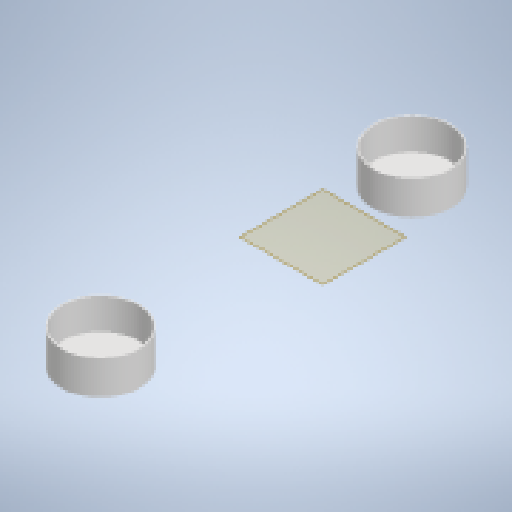
# Autodesk Inventor part: Base
Saved by Autodesk Inventor 2023.1 (Build 271208000, 208)
## iProperties
Created: 2023-07-08
Part Number: Base
Material: Generic
Document SubType Name: Modeling
Designer: Robot
Density: 1 g/cm^3
Appearance: Default
Author: Robot
Autodesk Inventor part; units mm, degrees
ref_plane "YZ Plane" through (0, 0, 0) normal (1, 0, 0) x (0, 1, 0)
ref_plane "XZ Plane" through (0, 0, 0) normal (0, 1, 0) x (-1, 0, 0)
ref_plane "XY Plane" through (0, 0, 0) normal (0, 0, 1) x (1, 0, 0)
ref_plane "Work Plane1" through (-8.7385, 18226.0351, -280.5199) normal (0, 1, 0) x (-0.9985279, 0, -0.0542412)
sketch "Sketch1" plane through (-8.7385, 18226.0351, -280.5199) normal (0, 1, 0) x (-0.9985279, 0, -0.0542412)
  circle A0 centre (-0.1598, -60.199) radius 25.4
  circle A1 centre (-0.1598, 150.601) radius 25.4
  circle A2 centre (-0.1598, 150.601) radius 26.4
  circle A3 centre (-0.1598, -60.199) radius 26.4
  line L0 (-17.3085, -5.3414) -> (16.6915, -5.3414)
  line L1 (16.6915, -5.3414) -> (16.6915, 52.8634)
  line L2 (16.6915, 52.8634) -> (-17.3085, 52.8634)
  line L3 (-17.3085, 52.8634) -> (-17.3085, -5.3414)
  line L4 (-17.3085, 52.8634) -> (-17.3085, 130.529)
  line L5 (-17.3085, -5.3414) -> (-17.3085, -40.1271)
  line L6 (16.6915, -5.3414) -> (16.6915, -39.8768)
  line L7 (16.6915, 52.8634) -> (16.6915, 130.2787)
  line L8 (31.4252, -66.238) -> (7.3835, -90.2796)
  line L9 (7.3835, -90.2796) -> (61.8308, -144.7269)
  line L10 (61.8308, -144.7269) -> (85.8724, -120.6852)
  line L11 (85.8724, -120.6852) -> (31.4252, -66.238)
  line L12 (30.0109, -67.6522) -> (84.4582, -122.0994)
  line L13 (8.7977, -88.8654) -> (63.245, -143.3126)
  line L14 (-6.1639, -91.881) -> (-30.2055, -67.8394)
  line L15 (-30.2055, -67.8394) -> (-84.6528, -122.2866)
  line L16 (-84.6528, -122.2866) -> (-60.6111, -146.3283)
  line L17 (-60.6111, -146.3283) -> (-6.1639, -91.881)
  line L18 (-7.5781, -90.4668) -> (-62.0253, -144.914)
  line L19 (-28.7913, -69.2536) -> (-83.2386, -123.7008)
  line L20 (84.9349, 211.9974) -> (60.8933, 236.039)
  line L21 (60.8933, 236.039) -> (6.446, 181.5918)
  line L22 (6.446, 181.5918) -> (30.4877, 157.5502)
  line L23 (30.4877, 157.5502) -> (84.9349, 211.9974)
  line L24 (83.5207, 213.4116) -> (29.0735, 158.9644)
  line L25 (62.3075, 234.6248) -> (7.8603, 180.1776)
  line L26 (-32.1213, 155.9317) -> (-8.0796, 179.9733)
  line L27 (-86.5685, 210.3789) -> (-32.1213, 155.9317)
  line L28 (-85.1543, 211.7931) -> (-30.707, 157.3459)
  line L29 (-62.5268, 234.4205) -> (-86.5685, 210.3789)
  line L30 (-63.9411, 233.0063) -> (-9.4938, 178.5591)
  line L31 (-8.0796, 179.9733) -> (-62.5268, 234.4205)
  line L32 (-7.5781, -90.4668) -> (-3.4984, -86.3871)
  line L33 (-6.1639, -91.881) -> (-0.8723, -86.5894)
  line L34 (-30.2055, -67.8394) -> (-26.295, -63.9289)
  line L35 (-28.7913, -69.2536) -> (-25.8437, -66.306)
  line L36 (31.4252, -66.238) -> (26.2268, -61.0397)
  line L37 (30.0109, -67.6522) -> (26.0131, -63.6544)
  line L38 (8.7977, -88.8654) -> (5.8404, -85.9081)
  line L39 (7.3835, -90.2796) -> (3.1788, -86.3871)
  line L40 (29.0735, 158.9644) -> (25.7539, 155.6448)
  line L41 (30.4877, 157.5502) -> (26.1142, 153.1768)
  line L42 (7.8603, 180.1776) -> (4.3036, 176.6209)
  line L43 (6.446, 181.5918) -> (1.7836, 176.9293)
  line L44 (-8.0796, 179.9733) -> (-4.7119, 176.6056)
  line L45 (-9.4938, 178.5591) -> (-7.0269, 176.0922)
  line L46 (-30.707, 157.3459) -> (-26.443, 153.0818)
  line L47 (-32.1213, 155.9317) -> (-26.5588, 150.3692)
  point P0 (-23.9414, 279.6329)
  point P1 (-30.2055, -67.8394)
  dimension "d3" = 52.8
  dimension "d4" = 52.8
  dimension "d0" = 50.8
  dimension "d1" = 50.8
  dimension "d2" = 210.8
  dimension "d9" = 34
  dimension "d18" = 34
  dimension "d19" = 77
  dimension "d20" = 2
  dimension "d21" = 2
  dimension "d22" = 34
  dimension "d23" = 77
  dimension "d24" = 2
  dimension "d25" = 2
  dimension "d26" = 34
  dimension "d27" = 77
  dimension "d28" = 2
  dimension "d29" = 2
  dimension "d30" = 34
  dimension "d31" = 77
  dimension "d32" = 2
  dimension "d33" = 2
  constraints: 96 end point, 21 parallel, 21 point on line, 15 perpendicular, 2 centre point, 2 coincident, 1 horizontal, 1 vertical, 24 other
  measures "d0" diameter of A0
  measures "d1" diameter of A1
  measures "d2" distance of A0.centre A1.centre
  measures "d9" distance between parallel lines of L1 L3
  measures "d18" distance between parallel lines of L9 L11
  measures "d19" distance between parallel lines of L10 L8
  measures "d20" distance between parallel lines of L12 L11
  measures "d21" distance between parallel lines of L9 L13
  measures "d22" distance between parallel lines of L15 L17
  measures "d23" distance between parallel lines of L16 L14
  measures "d24" distance between parallel lines of L18 L17
  measures "d25" distance between parallel lines of L15 L19
  measures "d26" distance between parallel lines of L21 L23
  measures "d27" distance between parallel lines of L22 L20
  measures "d28" distance between parallel lines of L24 L23
  measures "d29" distance between parallel lines of L21 L25
  measures "d30" distance between parallel lines of L27 L31
  measures "d31" distance between parallel lines of L26 L29
  measures "d32" distance between parallel lines of L30 L31
  measures "d33" distance between parallel lines of L27 L28
extrude "Extrusion1" add sketch "Sketch1" along normal blind 2 contours A0 | A1
extrude "Extrusion2" add sketch "Sketch1" along normal blind 23 contours A2 L26 | A3 | A2 L26
extrude "Extrusion3" add sketch "Sketch1" along normal blind 23 contours L7 L2 L4 A2 | L1 L0 L3 L2 | L6 A3 L5 L0
extrude "Extrusion4" add sketch "Sketch1" along normal blind 23 contours A2 L40 L22 L41 | L22 L24 L20 L23 | A2 L43 L22 L42 | L47 L26 L46 A2 | L22 L21 L20 L25 | L27 L29 L28 L26 | A2 L45 L26 L44 | L26 L30 L29 L31 | A3 L35 L14 L34 | L36 L8 L37 A3 | L14 L19 L16 L15 | L11 L10 L12 L8 | A3 L33 L14 L32 | L38 L8 L39 A3 | L14 L17 L16 L18 | L13 L10 L9 L8
sketch "Sketch2" plane through (-8.7385, 18249.0351, -280.5199) normal (0, 1, 0) x (0.9985279, 0, 0.0542412)
  line L0 (-83.5207, -213.4116) -> (-25.7539, -155.6448) projected
  arc A0 (-25.7539, -155.6448) -> (-4.3036, -176.6209) centre (0.1598, -150.601) ccw projected
  line L1 (-4.3036, -176.6209) -> (-62.3075, -234.6248) projected
  line L2 (63.9411, -233.0063) -> (7.0269, -176.0922) projected
  arc A1 (7.0269, -176.0922) -> (26.443, -153.0818) centre (0.1598, -150.601) ccw projected
  line L3 (26.443, -153.0818) -> (85.1543, -211.7931) projected
  line L4 (-26.0131, 63.6544) -> (-84.4582, 122.0994) projected
  arc A2 (-5.8404, 85.9081) -> (-26.0131, 63.6544) centre (0.1598, 60.199) ccw projected
  line L5 (-63.245, 143.3126) -> (-5.8404, 85.9081) projected
  line L6 (3.4984, 86.3871) -> (62.0253, 144.914) projected
  arc A3 (25.8437, 66.306) -> (3.4984, 86.3871) centre (0.1598, 60.199) ccw projected
  line L7 (83.2386, 123.7008) -> (25.8437, 66.306) projected
  line L8 (62.0253, 144.914) -> (83.2386, 123.7008)
  line L9 (-84.4582, 122.0994) -> (-85.8724, 120.6852) projected
  line L10 (-63.245, 143.3126) -> (-84.4582, 122.0994)
  line L11 (-4.3036, -176.6209) -> (-62.3075, -234.6248) projected
  line L12 (-62.3075, -234.6248) -> (-83.5207, -213.4116)
  line L13 (-83.5207, -213.4116) -> (-25.7539, -155.6448) projected
  line L14 (63.9411, -233.0063) -> (85.1543, -211.7931)
  point P0 (23.9414, -279.6329)
  point P1 (62.0253, 144.914)
  point P2 (-83.5207, -213.4116)
  constraints: 8 end point, 3 perpendicular, 2 point on line, 1 collinear
extrude "Extrusion5" add sketch "Sketch2" against normal blind 2
body "Solid1"
